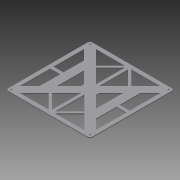
# Autodesk Inventor part: piastra_superiore_y
Saved by Autodesk Inventor 2014 SP1 (Build 180222100, 222)
## iProperties
Created: 2015-04-08
Part Number: piastra_superiore_y
Material: Generic
Document SubType Name: Modeling
Designer: Giorgio Nuzzo
Density: 1 g/cm^3
Appearance: Default
Author: Giorgio Nuzzo
Autodesk Inventor part; units mm, degrees
(part 1 of 3)
ref_plane "YZ Plane" through (0, 0, 0) normal (1, 0, 0) x (0, 1, 0)
ref_plane "XZ Plane" through (0, 0, 0) normal (0, 1, 0) x (-1, 0, 0)
ref_plane "XY Plane" through (0, 0, 0) normal (0, 0, 1) x (1, 0, 0)
sketch "Sketch1" plane through (0, 0, 0) normal (0, 0, 1) x (1, 0, 0)
  spline S0 degree 3 poles (-107.5002, -101.5001) (-107.5002, -104.8136) (-104.8138, -107.5001) (-101.5, -107.5001) knots 0 0 0 0 1 1 1 1
  line L0 (-107.5002, -101.5001) -> (-107.5002, -104.8136) construction
  line L1 (-107.5002, -104.8136) -> (-104.8138, -107.5001) construction
  line L2 (-104.8138, -107.5001) -> (-101.5, -107.5001) construction
  line L3 (-101.5, -107.5001) -> (101.5, -107.5001)
  spline S1 degree 3 poles (101.5, -107.5001) (104.8135, -107.5001) (107.5, -104.8136) (107.5, -101.5001) knots 2 2 2 2 3 3 3 3
  line L4 (101.5, -107.5001) -> (104.8135, -107.5001) construction
  line L5 (104.8135, -107.5001) -> (107.5, -104.8136) construction
  line L6 (107.5, -104.8136) -> (107.5, -101.5001) construction
  line L7 (107.5, -101.5001) -> (107.5, 101.5001)
  spline S2 degree 3 poles (107.5, 101.5001) (107.5, 104.8138) (104.8135, 107.5001) (101.5, 107.5001) (101.5, 107.5001) (-101.5, 107.5001) (-101.5, 107.5001) (-104.8138, 107.5001) (-107.5002, 104.8138) (-107.5002, 101.5001) (-107.5002, 101.5001) (-107.5002, -101.2971) (-107.5002, -101.5001) knots 4 4 4 4 5 5 5 6 6 6 7 7 7 8 8 8 8
  line L8 (107.5, 101.5001) -> (107.5, 104.8138) construction
  line L9 (107.5, 104.8138) -> (104.8135, 107.5001) construction
  line L10 (104.8135, 107.5001) -> (101.5, 107.5001) construction
  line L11 (101.5, 107.5001) -> (101.5, 107.5001) construction
  line L12 (101.5, 107.5001) -> (-101.5, 107.5001) construction
  line L13 (-101.5, 107.5001) -> (-101.5, 107.5001) construction
  line L14 (-101.5, 107.5001) -> (-104.8138, 107.5001) construction
  line L15 (-104.8138, 107.5001) -> (-107.5002, 104.8138) construction
  line L16 (-107.5002, 104.8138) -> (-107.5002, 101.5001) construction
  line L17 (-107.5002, 101.5001) -> (-107.5002, 101.5001) construction
  line L18 (-107.5002, 101.5001) -> (-107.5002, -101.5001) construction
  line L19 (-107.5002, -101.5001) -> (-107.5002, -101.5001) construction
  line L20 (4.9998, -107.5001) -> (84.925, -107.5001)
  line L21 (-97.4892, 82.4918) -> (-72.0064, 57.0089)
  line L22 (-72.0064, 57.0089) -> (-72.0064, 3.9999)
  line L23 (-72.0064, 3.9999) -> (-97.4892, 4.0106)
  line L24 (-97.4892, 4.0106) -> (-97.4892, 82.4918)
  line L25 (-97.4892, -82.4901) -> (-72.0064, -57.007)
  line L26 (-72.0064, -57.007) -> (-72.0064, -4.0001)
  line L27 (-72.0064, -4.0001) -> (-97.4892, -4.0001)
  line L28 (-97.4892, -4.0001) -> (-97.4892, -82.4901)
  line L29 (-19.4509, 4.4535) -> (-50.0063, 35.0089)
  line L30 (-50.0063, 35.0089) -> (-50.0063, -4.0001)
  line L31 (-50.0063, -4.0001) -> (-50.0063, -35.007)
  line L32 (-50.0063, -35.007) -> (-49.8928, -34.8936)
  line L33 (-49.8928, -34.8936) -> (-32.5743, -17.5752)
  line L34 (-32.5743, -17.5752) -> (-19.4509, -4.4518)
  line L35 (-19.4509, -4.4518) -> (-19.4509, -4.0001)
  line L36 (-19.4509, -4.0001) -> (-19.4509, 3.9999)
  line L37 (-19.4509, 3.9999) -> (-19.4509, 4.4535)
  line L38 (-3.9981, 93.318) -> (-3.9981, 18.9804)
  line L39 (-3.9981, 18.9804) -> (-32.5743, 47.5568)
  line L40 (-32.5743, 47.5568) -> (-41.1669, 56.1492)
  line L41 (-41.1669, 56.1492) -> (-3.9981, 93.318)
  line L42 (4.0017, 93.294) -> (41.1371, 56.1588)
  line L43 (41.1371, 56.1588) -> (4.0017, 19.0236)
  line L44 (4.0017, 19.0236) -> (4.0017, 93.294)
  line L45 (45.3797, 60.4015) -> (82.4876, 97.5093)
  line L46 (82.4876, 97.5093) -> (8.2719, 97.5093)
  line L47 (8.2719, 97.5093) -> (45.3797, 60.4015)
  line L48 (-8.2921, 97.5093) -> (-45.4095, 60.3918)
  line L49 (-45.4095, 60.3918) -> (-49.8928, 64.8751)
  line L50 (-49.8928, 64.8751) -> (-82.5268, 97.5093)
  line L51 (-82.5268, 97.5093) -> (-8.2921, 97.5093)
  line L52 (19.4003, -4.4028) -> (19.4003, -4.0001)
  line L53 (19.4003, -4.0001) -> (19.4003, 3.9999)
  line L54 (19.4003, 3.9999) -> (19.4003, 4.4423)
  line L55 (19.4003, 4.4423) -> (50.0062, 35.0482)
  line L56 (50.0062, 35.0482) -> (50.0062, 3.9999)
  line L57 (50.0062, 3.9999) -> (50.0062, -4.0001)
  line L58 (50.0062, -4.0001) -> (50.0062, -35.0087)
  line L59 (50.0062, -35.0087) -> (19.4003, -4.4028)
  line L60 (97.4996, 82.5416) -> (72.0062, 57.0482)
  line L61 (72.0062, 57.0482) -> (72.0062, 3.9999)
  line L62 (72.0062, 3.9999) -> (97.4996, 3.9999)
  line L63 (97.4996, 3.9999) -> (97.4996, 82.5416)
  line L64 (97.4996, -82.5021) -> (72.0062, -57.0088)
  line L65 (72.0062, -57.0088) -> (72.0062, -4.0001)
  line L66 (72.0062, -4.0001) -> (97.4996, -4.0001)
  line L67 (97.4996, -4.0001) -> (97.4996, -82.5021)
  line L68 (-8.2921, -97.3935) -> (-45.4095, -60.2761)
  line L69 (-45.4095, -60.2761) -> (-49.8928, -64.7595)
  line L70 (-49.8928, -64.7595) -> (-82.5268, -97.3935)
  line L71 (-82.5268, -97.3935) -> (-8.2921, -97.3935)
  line L72 (-3.9981, -93.2022) -> (-3.9981, -18.8647)
  line L73 (-3.9981, -18.8647) -> (-32.5743, -47.441)
  line L74 (-32.5743, -47.441) -> (-41.1669, -56.0334)
  line L75 (-41.1669, -56.0334) -> (-3.9981, -93.2022)
  line L76 (4.0017, -93.1785) -> (41.1371, -56.0431)
  line L77 (41.1371, -56.0431) -> (4.0017, -18.9081)
  line L78 (4.0017, -18.9081) -> (4.0017, -93.1785)
  line L79 (45.3797, -60.2857) -> (82.4876, -97.3935)
  line L80 (82.4876, -97.3935) -> (8.2719, -97.3935)
  line L81 (8.2719, -97.3935) -> (45.3797, -60.2857)
  line L82 (-102.0988, 0.0012) -> (-102.0907, 0.1648)
  line L83 (-102.0907, 0.1648) -> (-102.0664, 0.3237)
  line L84 (-102.0664, 0.3237) -> (-102.0269, 0.477)
  line L85 (-102.0269, 0.477) -> (-101.9732, 0.6241)
  line L86 (-101.9732, 0.6241) -> (-101.9057, 0.7639)
  line L87 (-101.9057, 0.7639) -> (-101.8256, 0.8957)
  line L88 (-101.8256, 0.8957) -> (-101.6302, 1.1326)
  line L89 (-101.6302, 1.1326) -> (-101.3934, 1.3279)
  line L90 (-101.3934, 1.3279) -> (-101.2614, 1.4082)
  line L91 (-101.2614, 1.4082) -> (-101.1216, 1.4755)
  line L92 (-101.1216, 1.4755) -> (-100.9746, 1.5293)
  line L93 (-100.9746, 1.5293) -> (-100.8213, 1.5687)
  line L94 (-100.8213, 1.5687) -> (-100.6625, 1.593)
  line L95 (-100.6625, 1.593) -> (-100.4989, 1.6013)
  line L96 (-100.4989, 1.6013) -> (-100.3352, 1.593)
  line L97 (-100.3352, 1.593) -> (-100.1764, 1.5687)
  line L98 (-100.1764, 1.5687) -> (-100.0231, 1.5293)
  line L99 (-100.0231, 1.5293) -> (-99.876, 1.4755)
  line L100 (-99.876, 1.4755) -> (-99.7361, 1.4082)
  line L101 (-99.7361, 1.4082) -> (-99.6043, 1.3279)
  line L102 (-99.6043, 1.3279) -> (-99.3675, 1.1326)
  line L103 (-99.3675, 1.1326) -> (-99.1722, 0.8957)
  line L104 (-99.1722, 0.8957) -> (-99.0919, 0.7639)
  line L105 (-99.0919, 0.7639) -> (-99.0245, 0.6241)
  line L106 (-99.0245, 0.6241) -> (-98.9708, 0.477)
  line L107 (-98.9708, 0.477) -> (-98.9313, 0.3237)
  line L108 (-98.9313, 0.3237) -> (-98.9071, 0.1648)
  line L109 (-98.9071, 0.1648) -> (-98.8988, 0.0012)
  line L110 (-98.8988, 0.0012) -> (-98.9071, -0.1624)
  line L111 (-98.9071, -0.1624) -> (-98.9313, -0.3213)
  line L112 (-98.9313, -0.3213) -> (-98.9708, -0.4747)
  line L113 (-98.9708, -0.4747) -> (-99.0245, -0.6215)
  line L114 (-99.0245, -0.6215) -> (-99.0919, -0.7614)
  line L115 (-99.0919, -0.7614) -> (-99.1722, -0.8933)
  line L116 (-99.1722, -0.8933) -> (-99.3675, -1.13)
  line L117 (-99.3675, -1.13) -> (-99.6043, -1.3257)
  line L118 (-99.6043, -1.3257) -> (-99.7361, -1.4056)
  line L119 (-99.7361, -1.4056) -> (-99.876, -1.4731)
  line L120 (-99.876, -1.4731) -> (-100.0231, -1.5269)
  line L121 (-100.0231, -1.5269) -> (-100.1764, -1.5661)
  line L122 (-100.1764, -1.5661) -> (-100.3352, -1.5906)
  line L123 (-100.3352, -1.5906) -> (-100.4989, -1.5989)
  line L124 (-100.4989, -1.5989) -> (-100.6625, -1.5906)
  line L125 (-100.6625, -1.5906) -> (-100.8213, -1.5661)
  line L126 (-100.8213, -1.5661) -> (-100.9746, -1.5269)
  line L127 (-100.9746, -1.5269) -> (-101.1216, -1.4731)
  line L128 (-101.1216, -1.4731) -> (-101.2614, -1.4056)
  line L129 (-101.2614, -1.4056) -> (-101.3934, -1.3257)
  line L130 (-101.3934, -1.3257) -> (-101.6302, -1.13)
  line L131 (-101.6302, -1.13) -> (-101.8256, -0.8933)
  line L132 (-101.8256, -0.8933) -> (-101.9057, -0.7614)
  line L133 (-101.9057, -0.7614) -> (-101.9732, -0.6215)
  line L134 (-101.9732, -0.6215) -> (-102.0269, -0.4747)
  line L135 (-102.0269, -0.4747) -> (-102.0664, -0.3213)
  line L136 (-102.0664, -0.3213) -> (-102.0907, -0.1624)
  line L137 (-102.0907, -0.1624) -> (-102.0988, 0.0012)
  line L138 (98.899, 0.0012) -> (98.9072, 0.1648)
  line L139 (98.9072, 0.1648) -> (98.9317, 0.3237)
  line L140 (98.9317, 0.3237) -> (98.971, 0.477)
  line L141 (98.971, 0.477) -> (99.0247, 0.6241)
  line L142 (99.0247, 0.6241) -> (99.0922, 0.7639)
  line L143 (99.0922, 0.7639) -> (99.1725, 0.8957)
  line L144 (99.1725, 0.8957) -> (99.3678, 1.1326)
  line L145 (99.3678, 1.1326) -> (99.6045, 1.3279)
  line L146 (99.6045, 1.3279) -> (99.7365, 1.4082)
  line L147 (99.7365, 1.4082) -> (99.8763, 1.4755)
  line L148 (99.8763, 1.4755) -> (100.0234, 1.5293)
  line L149 (100.0234, 1.5293) -> (100.1767, 1.5687)
  line L150 (100.1767, 1.5687) -> (100.3356, 1.593)
  line L151 (100.3356, 1.593) -> (100.4992, 1.6013)
  line L152 (100.4992, 1.6013) -> (100.6628, 1.593)
  line L153 (100.6628, 1.593) -> (100.8217, 1.5687)
  line L154 (100.8217, 1.5687) -> (100.975, 1.5293)
  line L155 (100.975, 1.5293) -> (101.1217, 1.4755)
  line L156 (101.1217, 1.4755) -> (101.2616, 1.4082)
  line L157 (101.2616, 1.4082) -> (101.3936, 1.3279)
  line L158 (101.3936, 1.3279) -> (101.6306, 1.1326)
  line L159 (101.6306, 1.1326) -> (101.8259, 0.8957)
  line L160 (101.8259, 0.8957) -> (101.9058, 0.7639)
  line L161 (101.9058, 0.7639) -> (101.9734, 0.6241)
  line L162 (101.9734, 0.6241) -> (102.0271, 0.477)
  line L163 (102.0271, 0.477) -> (102.0667, 0.3237)
  line L164 (102.0667, 0.3237) -> (102.0908, 0.1648)
  line L165 (102.0908, 0.1648) -> (102.0991, 0.0012)
  line L166 (102.0991, 0.0012) -> (102.0908, -0.1624)
  line L167 (102.0908, -0.1624) -> (102.0667, -0.3213)
  line L168 (102.0667, -0.3213) -> (102.0271, -0.4747)
  line L169 (102.0271, -0.4747) -> (101.9734, -0.6215)
  line L170 (101.9734, -0.6215) -> (101.9058, -0.7614)
  line L171 (101.9058, -0.7614) -> (101.8259, -0.8933)
  line L172 (101.8259, -0.8933) -> (101.6306, -1.13)
  line L173 (101.6306, -1.13) -> (101.3936, -1.3257)
  line L174 (101.3936, -1.3257) -> (101.2616, -1.4056)
  line L175 (101.2616, -1.4056) -> (101.1217, -1.4731)
  line L176 (101.1217, -1.4731) -> (100.975, -1.5269)
  line L177 (100.975, -1.5269) -> (100.8217, -1.5661)
  line L178 (100.8217, -1.5661) -> (100.6628, -1.5906)
  line L179 (100.6628, -1.5906) -> (100.4992, -1.5989)
  line L180 (100.4992, -1.5989) -> (100.3356, -1.5906)
  line L181 (100.3356, -1.5906) -> (100.1767, -1.5661)
  line L182 (100.1767, -1.5661) -> (100.0234, -1.5269)
  line L183 (100.0234, -1.5269) -> (99.8763, -1.4731)
  line L184 (99.8763, -1.4731) -> (99.7365, -1.4056)
  line L185 (99.7365, -1.4056) -> (99.6045, -1.3257)
  line L186 (99.6045, -1.3257) -> (99.3678, -1.13)
  line L187 (99.3678, -1.13) -> (99.1725, -0.8933)
  line L188 (99.1725, -0.8933) -> (99.0922, -0.7614)
  line L189 (99.0922, -0.7614) -> (99.0247, -0.6215)
  line L190 (99.0247, -0.6215) -> (98.971, -0.4747)
  line L191 (98.971, -0.4747) -> (98.9317, -0.3213)
  line L192 (98.9317, -0.3213) -> (98.9072, -0.1624)
  line L193 (98.9072, -0.1624) -> (98.899, 0.0012)
  line L194 (-1.6014, 100.496) -> (-1.5931, 100.6595)
  line L195 (-1.5931, 100.6595) -> (-1.5688, 100.8185)
  line L196 (-1.5688, 100.8185) -> (-1.5294, 100.9718)
  line L197 (-1.5294, 100.9718) -> (-1.4756, 101.1187)
  line L198 (-1.4756, 101.1187) -> (-1.4083, 101.2586)
  line L199 (-1.4083, 101.2586) -> (-1.328, 101.3905)
  line L200 (-1.328, 101.3905) -> (-1.1327, 101.6274)
  line L201 (-1.1327, 101.6274) -> (-0.8958, 101.8227)
  line L202 (-0.8958, 101.8227) -> (-0.764, 101.9028)
  line L203 (-0.764, 101.9028) -> (-0.6242, 101.9702)
  line L204 (-0.6242, 101.9702) -> (-0.4771, 102.0241)
  line L205 (-0.4771, 102.0241) -> (-0.3238, 102.0634)
  line L206 (-0.3238, 102.0634) -> (-0.1649, 102.0877)
  line L207 (-0.1649, 102.0877) -> (-0.0013, 102.0959)
  line L208 (-0.0013, 102.0959) -> (0.1622, 102.0877)
  line L209 (0.1622, 102.0877) -> (0.321, 102.0634)
  line L210 (0.321, 102.0634) -> (0.4746, 102.0241)
  line L211 (0.4746, 102.0241) -> (0.6214, 101.9702)
  line L212 (0.6214, 101.9702) -> (0.7613, 101.9028)
  line L213 (0.7613, 101.9028) -> (0.8932, 101.8227)
  line L214 (0.8932, 101.8227) -> (1.1299, 101.6274)
  line L215 (1.1299, 101.6274) -> (1.3256, 101.3905)
  line L216 (1.3256, 101.3905) -> (1.4055, 101.2586)
  line L217 (1.4055, 101.2586) -> (1.473, 101.1187)
  line L218 (1.473, 101.1187) -> (1.5268, 100.9718)
  line L219 (1.5268, 100.9718) -> (1.5661, 100.8185)
  line L220 (1.5661, 100.8185) -> (1.5905, 100.6595)
  line L221 (1.5905, 100.6595) -> (1.5988, 100.496)
  line L222 (1.5988, 100.496) -> (1.5905, 100.3324)
  line L223 (1.5905, 100.3324) -> (1.5661, 100.1736)
  line L224 (1.5661, 100.1736) -> (1.5268, 100.0201)
  line L225 (1.5268, 100.0201) -> (1.473, 99.8731)
  line L226 (1.473, 99.8731) -> (1.4055, 99.7333)
  line L227 (1.4055, 99.7333) -> (1.3256, 99.6013)
  line L228 (1.3256, 99.6013) -> (1.1299, 99.3646)
  line L229 (1.1299, 99.3646) -> (0.8932, 99.1691)
  line L230 (0.8932, 99.1691) -> (0.7613, 99.089)
  line L231 (0.7613, 99.089) -> (0.6214, 99.0217)
  line L232 (0.6214, 99.0217) -> (0.4746, 98.9679)
  line L233 (0.4746, 98.9679) -> (0.321, 98.9285)
  line L234 (0.321, 98.9285) -> (0.1622, 98.9042)
  line L235 (0.1622, 98.9042) -> (-0.0013, 98.8959)
  line L236 (-0.0013, 98.8959) -> (-0.1649, 98.9042)
  line L237 (-0.1649, 98.9042) -> (-0.3238, 98.9285)
  line L238 (-0.3238, 98.9285) -> (-0.4771, 98.9679)
  line L239 (-0.4771, 98.9679) -> (-0.6242, 99.0217)
  line L240 (-0.6242, 99.0217) -> (-0.764, 99.089)
  line L241 (-0.764, 99.089) -> (-0.8958, 99.1691)
  line L242 (-0.8958, 99.1691) -> (-1.1327, 99.3646)
  line L243 (-1.1327, 99.3646) -> (-1.328, 99.6013)
  line L244 (-1.328, 99.6013) -> (-1.4083, 99.7333)
  line L245 (-1.4083, 99.7333) -> (-1.4756, 99.8731)
  line L246 (-1.4756, 99.8731) -> (-1.5294, 100.0201)
  line L247 (-1.5294, 100.0201) -> (-1.5688, 100.1736)
  line L248 (-1.5688, 100.1736) -> (-1.5931, 100.3324)
  line L249 (-1.5931, 100.3324) -> (-1.6014, 100.496)
  line L250 (-1.6014, -100.4996) -> (-1.5931, -100.336)
  line L251 (-1.5931, -100.336) -> (-1.5688, -100.1772)
  line L252 (-1.5688, -100.1772) -> (-1.5294, -100.0239)
  line L253 (-1.5294, -100.0239) -> (-1.4756, -99.8768)
  line L254 (-1.4756, -99.8768) -> (-1.4083, -99.7369)
  line L255 (-1.4083, -99.7369) -> (-1.328, -99.6049)
  line L256 (-1.328, -99.6049) -> (-1.1327, -99.3683)
  line L257 (-1.1327, -99.3683) -> (-0.8958, -99.1729)
  line L258 (-0.8958, -99.1729) -> (-0.764, -99.0927)
  line L259 (-0.764, -99.0927) -> (-0.6242, -99.0255)
  line L260 (-0.6242, -99.0255) -> (-0.4771, -98.9717)
  line L261 (-0.4771, -98.9717) -> (-0.3238, -98.9321)
  line L262 (-0.3238, -98.9321) -> (-0.1649, -98.908)
  line L263 (-0.1649, -98.908) -> (-0.0013, -98.8997)
  line L264 (-0.0013, -98.8997) -> (0.1622, -98.908)
  line L265 (0.1622, -98.908) -> (0.321, -98.9321)
  line L266 (0.321, -98.9321) -> (0.4746, -98.9717)
  line L267 (0.4746, -98.9717) -> (0.6214, -99.0255)
  line L268 (0.6214, -99.0255) -> (0.7613, -99.0927)
  line L269 (0.7613, -99.0927) -> (0.8932, -99.1729)
  line L270 (0.8932, -99.1729) -> (1.1299, -99.3683)
  line L271 (1.1299, -99.3683) -> (1.3256, -99.6049)
  line L272 (1.3256, -99.6049) -> (1.4055, -99.7369)
  line L273 (1.4055, -99.7369) -> (1.473, -99.8768)
  line L274 (1.473, -99.8768) -> (1.5268, -100.0239)
  line L275 (1.5268, -100.0239) -> (1.5661, -100.1772)
  line L276 (1.5661, -100.1772) -> (1.5905, -100.336)
  line L277 (1.5905, -100.336) -> (1.5988, -100.4996)
  line L278 (1.5988, -100.4996) -> (1.5905, -100.6633)
  line L279 (1.5905, -100.6633) -> (1.5661, -100.8221)
  line L280 (1.5661, -100.8221) -> (1.5268, -100.9754)
  line L281 (1.5268, -100.9754) -> (1.473, -101.1225)
  line L282 (1.473, -101.1225) -> (1.4055, -101.2624)
  line L283 (1.4055, -101.2624) -> (1.3256, -101.3943)
  line L284 (1.3256, -101.3943) -> (1.1299, -101.631)
  line L285 (1.1299, -101.631) -> (0.8932, -101.8263)
  line L286 (0.8932, -101.8263) -> (0.7613, -101.9066)
  line L287 (0.7613, -101.9066) -> (0.6214, -101.9738)
  line L288 (0.6214, -101.9738) -> (0.4746, -102.0279)
  line L289 (0.4746, -102.0279) -> (0.321, -102.0672)
  line L290 (0.321, -102.0672) -> (0.1622, -102.0913)
  line L291 (0.1622, -102.0913) -> (-0.0013, -102.0995)
  line L292 (-0.0013, -102.0995) -> (-0.1649, -102.0913)
  line L293 (-0.1649, -102.0913) -> (-0.3238, -102.0672)
  line L294 (-0.3238, -102.0672) -> (-0.4771, -102.0279)
  line L295 (-0.4771, -102.0279) -> (-0.6242, -101.9738)
  line L296 (-0.6242, -101.9738) -> (-0.764, -101.9066)
  line L297 (-0.764, -101.9066) -> (-0.8958, -101.8263)
  line L298 (-0.8958, -101.8263) -> (-1.1327, -101.631)
  line L299 (-1.1327, -101.631) -> (-1.328, -101.3943)
  line L300 (-1.328, -101.3943) -> (-1.4083, -101.2624)
  line L301 (-1.4083, -101.2624) -> (-1.4756, -101.1225)
  line L302 (-1.4756, -101.1225) -> (-1.5294, -100.9754)
  line L303 (-1.5294, -100.9754) -> (-1.5688, -100.8221)
  line L304 (-1.5688, -100.8221) -> (-1.5931, -100.6633)
  line L305 (-1.5931, -100.6633) -> (-1.6014, -100.4996)
  line L306 (98.899, -100.5) -> (98.9072, -100.3363)
  line L307 (98.9072, -100.3363) -> (98.9313, -100.1775)
  line L308 (98.9313, -100.1775) -> (98.971, -100.0242)
  line L309 (98.971, -100.0242) -> (99.0247, -99.8771)
  line L310 (99.0247, -99.8771) -> (99.0919, -99.7372)
  line L311 (99.0919, -99.7372) -> (99.1722, -99.6053)
  line L312 (99.1722, -99.6053) -> (99.3675, -99.3686)
  line L313 (99.3675, -99.3686) -> (99.6045, -99.1733)
  line L314 (99.6045, -99.1733) -> (99.7361, -99.093)
  line L315 (99.7361, -99.093) -> (99.876, -99.0258)
  line L316 (99.876, -99.0258) -> (100.0231, -98.9721)
  line L317 (100.0231, -98.9721) -> (100.1764, -98.9325)
  line L318 (100.1764, -98.9325) -> (100.3352, -98.9083)
  line L319 (100.3352, -98.9083) -> (100.4989, -98.9001)
  line L320 (100.4989, -98.9001) -> (100.6625, -98.9083)
  line L321 (100.6625, -98.9083) -> (100.8213, -98.9325)
  line L322 (100.8213, -98.9325) -> (100.9746, -98.9721)
  line L323 (100.9746, -98.9721) -> (101.1217, -99.0258)
  line L324 (101.1217, -99.0258) -> (101.2616, -99.093)
  line L325 (101.2616, -99.093) -> (101.3936, -99.1733)
  line L326 (101.3936, -99.1733) -> (101.6302, -99.3686)
  line L327 (101.6302, -99.3686) -> (101.8256, -99.6053)
  line L328 (101.8256, -99.6053) -> (101.9058, -99.7372)
  line L329 (101.9058, -99.7372) -> (101.973, -99.8771)
  line L330 (101.973, -99.8771) -> (102.0271, -100.0242)
  line L331 (102.0271, -100.0242) -> (102.0664, -100.1775)
  line L332 (102.0664, -100.1775) -> (102.0905, -100.3363)
  line L333 (102.0905, -100.3363) -> (102.0988, -100.5)
  line L334 (102.0988, -100.5) -> (102.0905, -100.6636)
  line L335 (102.0905, -100.6636) -> (102.0664, -100.8224)
  line L336 (102.0664, -100.8224) -> (102.0271, -100.9757)
  line L337 (102.0271, -100.9757) -> (101.973, -101.1229)
  line L338 (101.973, -101.1229) -> (101.9058, -101.2627)
  line L339 (101.9058, -101.2627) -> (101.8256, -101.3947)
  line L340 (101.8256, -101.3947) -> (101.6302, -101.6314)
  line L341 (101.6302, -101.6314) -> (101.3936, -101.8267)
  line L342 (101.3936, -101.8267) -> (101.2616, -101.907)
  line L343 (101.2616, -101.907) -> (101.1217, -101.9741)
  line L344 (101.1217, -101.9741) -> (100.9746, -102.0282)
  line L345 (100.9746, -102.0282) -> (100.8213, -102.0675)
  line L346 (100.8213, -102.0675) -> (100.6625, -102.0916)
  line L347 (100.6625, -102.0916) -> (100.4989, -102.0999)
  line L348 (100.4989, -102.0999) -> (100.3352, -102.0916)
  line L349 (100.3352, -102.0916) -> (100.1764, -102.0675)
  line L350 (100.1764, -102.0675) -> (100.0231, -102.0282)
  line L351 (100.0231, -102.0282) -> (99.876, -101.9741)
  line L352 (99.876, -101.9741) -> (99.7361, -101.907)
  line L353 (99.7361, -101.907) -> (99.6045, -101.8267)
  line L354 (99.6045, -101.8267) -> (99.3675, -101.6314)
  line L355 (99.3675, -101.6314) -> (99.1722, -101.3947)
  line L356 (99.1722, -101.3947) -> (99.0919, -101.2627)
  line L357 (99.0919, -101.2627) -> (99.0247, -101.1229)
  line L358 (99.0247, -101.1229) -> (98.971, -100.9757)
  line L359 (98.971, -100.9757) -> (98.9313, -100.8224)
  line L360 (98.9313, -100.8224) -> (98.9072, -100.6636)
  line L361 (98.9072, -100.6636) -> (98.899, -100.5)
  line L362 (-102.1177, -100.4983) -> (-102.1094, -100.3346)
  line L363 (-102.1094, -100.3346) -> (-102.0852, -100.1758)
  line L364 (-102.0852, -100.1758) -> (-102.0457, -100.0225)
  line L365 (-102.0457, -100.0225) -> (-101.992, -99.8754)
  line L366 (-101.992, -99.8754) -> (-101.9246, -99.7355)
  line L367 (-101.9246, -99.7355) -> (-101.8443, -99.6036)
  line L368 (-101.8443, -99.6036) -> (-101.649, -99.3669)
  line L369 (-101.649, -99.3669) -> (-101.4122, -99.1716)
  line L370 (-101.4122, -99.1716) -> (-101.2804, -99.0913)
  line L371 (-101.2804, -99.0913) -> (-101.1405, -99.0241)
  line L372 (-101.1405, -99.0241) -> (-100.9934, -98.97)
  line L373 (-100.9934, -98.97) -> (-100.8401, -98.9307)
  line L374 (-100.8401, -98.9307) -> (-100.6813, -98.9066)
  line L375 (-100.6813, -98.9066) -> (-100.5176, -98.8984)
  line L376 (-100.5176, -98.8984) -> (-100.354, -98.9066)
  line L377 (-100.354, -98.9066) -> (-100.1952, -98.9307)
  line L378 (-100.1952, -98.9307) -> (-100.0419, -98.97)
  line L379 (-100.0419, -98.97) -> (-99.8949, -99.0241)
  line L380 (-99.8949, -99.0241) -> (-99.7551, -99.0913)
  line L381 (-99.7551, -99.0913) -> (-99.6231, -99.1716)
  line L382 (-99.6231, -99.1716) -> (-99.3863, -99.3669)
  line L383 (-99.3863, -99.3669) -> (-99.1909, -99.6036)
  line L384 (-99.1909, -99.6036) -> (-99.1108, -99.7355)
  line L385 (-99.1108, -99.7355) -> (-99.0433, -99.8754)
  line L386 (-99.0433, -99.8754) -> (-98.9896, -100.0225)
  line L387 (-98.9896, -100.0225) -> (-98.9501, -100.1758)
  line L388 (-98.9501, -100.1758) -> (-98.9258, -100.3346)
  line L389 (-98.9258, -100.3346) -> (-98.9176, -100.4983)
  line L390 (-98.9176, -100.4983) -> (-98.9258, -100.6619)
  line L391 (-98.9258, -100.6619) -> (-98.9501, -100.8207)
  line L392 (-98.9501, -100.8207) -> (-98.9896, -100.974)
  line L393 (-98.9896, -100.974) -> (-99.0433, -101.1211)
  line L394 (-99.0433, -101.1211) -> (-99.1108, -101.261)
  line L395 (-99.1108, -101.261) -> (-99.1909, -101.3929)
  line L396 (-99.1909, -101.3929) -> (-99.3863, -101.6296)
  line L397 (-99.3863, -101.6296) -> (-99.6231, -101.825)
  line L398 (-99.6231, -101.825) -> (-99.7551, -101.9052)
  line L399 (-99.7551, -101.9052) -> (-99.8949, -101.9724)
  line L400 (-99.8949, -101.9724) -> (-100.0419, -102.0262)
  line L401 (-100.0419, -102.0262) -> (-100.1952, -102.0658)
  line L402 (-100.1952, -102.0658) -> (-100.354, -102.0899)
  line L403 (-100.354, -102.0899) -> (-100.5176, -102.0982)
  line L404 (-100.5176, -102.0982) -> (-100.6813, -102.0899)
  line L405 (-100.6813, -102.0899) -> (-100.8401, -102.0658)
  line L406 (-100.8401, -102.0658) -> (-100.9934, -102.0262)
  line L407 (-100.9934, -102.0262) -> (-101.1405, -101.9724)
  line L408 (-101.1405, -101.9724) -> (-101.2804, -101.9052)
  line L409 (-101.2804, -101.9052) -> (-101.4122, -101.825)
  line L410 (-101.4122, -101.825) -> (-101.649, -101.6296)
  line L411 (-101.649, -101.6296) -> (-101.8443, -101.3929)
  line L412 (-101.8443, -101.3929) -> (-101.9246, -101.261)
  line L413 (-101.9246, -101.261) -> (-101.992, -101.1211)
  line L414 (-101.992, -101.1211) -> (-102.0457, -100.974)
  line L415 (-102.0457, -100.974) -> (-102.0852, -100.8207)
  line L416 (-102.0852, -100.8207) -> (-102.1094, -100.6619)
  line L417 (-102.1094, -100.6619) -> (-102.1177, -100.4983)
  line L418 (-102.1001, 100.5) -> (-102.0919, 100.6636)
  line L419 (-102.0919, 100.6636) -> (-102.0676, 100.8224)
  line L420 (-102.0676, 100.8224) -> (-102.0281, 100.9757)
  line L421 (-102.0281, 100.9757) -> (-101.9744, 101.1229)
  line L422 (-101.9744, 101.1229) -> (-101.907, 101.2627)
  line L423 (-101.907, 101.2627) -> (-101.8268, 101.3945)
  line L424 (-101.8268, 101.3945) -> (-101.6314, 101.6314)
  line L425 (-101.6314, 101.6314) -> (-101.3946, 101.8267)
  line L426 (-101.3946, 101.8267) -> (-101.2628, 101.907)
  line L427 (-101.2628, 101.907) -> (-101.1229, 101.9743)
  line L428 (-101.1229, 101.9743) -> (-100.9758, 102.0281)
  line L429 (-100.9758, 102.0281) -> (-100.8225, 102.0675)
  line L430 (-100.8225, 102.0675) -> (-100.6637, 102.0918)
  line L431 (-100.6637, 102.0918) -> (-100.5001, 102.1001)
  line L432 (-100.5001, 102.1001) -> (-100.3364, 102.0918)
  line L433 (-100.3364, 102.0918) -> (-100.1776, 102.0675)
  line L434 (-100.1776, 102.0675) -> (-100.0243, 102.0281)
  line L435 (-100.0243, 102.0281) -> (-99.8774, 101.9743)
  line L436 (-99.8774, 101.9743) -> (-99.7375, 101.907)
  line L437 (-99.7375, 101.907) -> (-99.6055, 101.8267)
  line L438 (-99.6055, 101.8267) -> (-99.3687, 101.6314)
  line L439 (-99.3687, 101.6314) -> (-99.1734, 101.3945)
  line L440 (-99.1734, 101.3945) -> (-99.0933, 101.2627)
  line L441 (-99.0933, 101.2627) -> (-99.0257, 101.1229)
  line L442 (-99.0257, 101.1229) -> (-98.972, 100.9757)
  line L443 (-98.972, 100.9757) -> (-98.9325, 100.8224)
  line L444 (-98.9325, 100.8224) -> (-98.9084, 100.6636)
  line L445 (-98.9084, 100.6636) -> (-98.9002, 100.5)
  line L446 (-98.9002, 100.5) -> (-98.9084, 100.3363)
  line L447 (-98.9084, 100.3363) -> (-98.9325, 100.1775)
  line L448 (-98.9325, 100.1775) -> (-98.972, 100.0242)
  line L449 (-98.972, 100.0242) -> (-99.0257, 99.8773)
  line L450 (-99.0257, 99.8773) -> (-99.0933, 99.7374)
  line L451 (-99.0933, 99.7374) -> (-99.1734, 99.6055)
  line L452 (-99.1734, 99.6055) -> (-99.3687, 99.3686)
  line L453 (-99.3687, 99.3686) -> (-99.6055, 99.1733)
  line L454 (-99.6055, 99.1733) -> (-99.7375, 99.0932)
  line L455 (-99.7375, 99.0932) -> (-99.8774, 99.0258)
  line L456 (-99.8774, 99.0258) -> (-100.0243, 98.9719)
  line L457 (-100.0243, 98.9719) -> (-100.1776, 98.9325)
  line L458 (-100.1776, 98.9325) -> (-100.3364, 98.9083)
  line L459 (-100.3364, 98.9083) -> (-100.5001, 98.9001)
  line L460 (-100.5001, 98.9001) -> (-100.6637, 98.9083)
  line L461 (-100.6637, 98.9083) -> (-100.8225, 98.9325)
  line L462 (-100.8225, 98.9325) -> (-100.9758, 98.9719)
  line L463 (-100.9758, 98.9719) -> (-101.1229, 99.0258)
  line L464 (-101.1229, 99.0258) -> (-101.2628, 99.0932)
  line L465 (-101.2628, 99.0932) -> (-101.3946, 99.1733)
  line L466 (-101.3946, 99.1733) -> (-101.6314, 99.3686)
  line L467 (-101.6314, 99.3686) -> (-101.8268, 99.6055)
  line L468 (-101.8268, 99.6055) -> (-101.907, 99.7374)
  line L469 (-101.907, 99.7374) -> (-101.9744, 99.8773)
  line L470 (-101.9744, 99.8773) -> (-102.0281, 100.0242)
  line L471 (-102.0281, 100.0242) -> (-102.0676, 100.1775)
  line L472 (-102.0676, 100.1775) -> (-102.0919, 100.3363)
  line L473 (-102.0919, 100.3363) -> (-102.1001, 100.5)
  line L474 (98.9003, 100.5) -> (98.9086, 100.6636)
  line L475 (98.9086, 100.6636) -> (98.9327, 100.8224)
  line L476 (98.9327, 100.8224) -> (98.972, 100.9757)
  line L477 (98.972, 100.9757) -> (99.0261, 101.1229)
  line L478 (99.0261, 101.1229) -> (99.0933, 101.2627)
  line L479 (99.0933, 101.2627) -> (99.1735, 101.3945)
  line L480 (99.1735, 101.3945) -> (99.3689, 101.6314)
  line L481 (99.3689, 101.6314) -> (99.6055, 101.8267)
  line L482 (99.6055, 101.8267) -> (99.7375, 101.907)
  line L483 (99.7375, 101.907) -> (99.8774, 101.9743)
  line L484 (99.8774, 101.9743) -> (100.0245, 102.0281)
  line L485 (100.0245, 102.0281) -> (100.1778, 102.0675)
  line L486 (100.1778, 102.0675) -> (100.3366, 102.0918)
  line L487 (100.3366, 102.0918) -> (100.5002, 102.1001)
  line L488 (100.5002, 102.1001) -> (100.6639, 102.0918)
  line L489 (100.6639, 102.0918) -> (100.8227, 102.0675)
  line L490 (100.8227, 102.0675) -> (100.976, 102.0281)
  line L491 (100.976, 102.0281) -> (101.1231, 101.9743)
  line L492 (101.1231, 101.9743) -> (101.263, 101.907)
  line L493 (101.263, 101.907) -> (101.3949, 101.8267)
  line L494 (101.3949, 101.8267) -> (101.6316, 101.6314)
  line L495 (101.6316, 101.6314) -> (101.8269, 101.3945)
  line L496 (101.8269, 101.3945) -> (101.9072, 101.2627)
  line L497 (101.9072, 101.2627) -> (101.9744, 101.1229)
  line L498 (101.9744, 101.1229) -> (102.0281, 100.9757)
  line L499 (102.0281, 100.9757) -> (102.0678, 100.8224)
  line L500 (102.0678, 100.8224) -> (102.0919, 100.6636)
  line L501 (102.0919, 100.6636) -> (102.1001, 100.5)
  line L502 (102.1001, 100.5) -> (102.0919, 100.3363)
  line L503 (102.0919, 100.3363) -> (102.0678, 100.1775)
  line L504 (102.0678, 100.1775) -> (102.0281, 100.0242)
  line L505 (102.0281, 100.0242) -> (101.9744, 99.8773)
  line L506 (101.9744, 99.8773) -> (101.9072, 99.7374)
  line L507 (101.9072, 99.7374) -> (101.8269, 99.6055)
  line L508 (101.8269, 99.6055) -> (101.6316, 99.3686)
  line L509 (101.6316, 99.3686) -> (101.3949, 99.1733)
  line L510 (101.3949, 99.1733) -> (101.263, 99.0932)
  line L511 (101.263, 99.0932) -> (101.1231, 99.0258)
  line L512 (101.1231, 99.0258) -> (100.976, 98.9719)
  line L513 (100.976, 98.9719) -> (100.8227, 98.9325)
  line L514 (100.8227, 98.9325) -> (100.6639, 98.9083)
  line L515 (100.6639, 98.9083) -> (100.5002, 98.9001)
  line L516 (100.5002, 98.9001) -> (100.3366, 98.9083)
  line L517 (100.3366, 98.9083) -> (100.1778, 98.9325)
  line L518 (100.1778, 98.9325) -> (100.0245, 98.9719)
  line L519 (100.0245, 98.9719) -> (99.8774, 99.0258)
  line L520 (99.8774, 99.0258) -> (99.7375, 99.0932)
  line L521 (99.7375, 99.0932) -> (99.6055, 99.1733)
  line L522 (99.6055, 99.1733) -> (99.3689, 99.3686)
  line L523 (99.3689, 99.3686) -> (99.1735, 99.6055)
  line L524 (99.1735, 99.6055) -> (99.0933, 99.7374)
  line L525 (99.0933, 99.7374) -> (99.0261, 99.8773)
  line L526 (99.0261, 99.8773) -> (98.972, 100.0242)
  line L527 (98.972, 100.0242) -> (98.9327, 100.1775)
  line L528 (98.9327, 100.1775) -> (98.9086, 100.3363)
  line L529 (98.9086, 100.3363) -> (98.9003, 100.5)
  line L530 (76.8948, 78.513) -> (76.9031, 78.6767)
  line L531 (76.9031, 78.6767) -> (76.9272, 78.8355)
  line L532 (76.9272, 78.8355) -> (76.9668, 78.9888)
  line L533 (76.9668, 78.9888) -> (77.0205, 79.1359)
  line L534 (77.0205, 79.1359) -> (77.0877, 79.2758)
  line L535 (77.0877, 79.2758) -> (77.168, 79.4076)
  line L536 (77.168, 79.4076) -> (77.3633, 79.6444)
  line L537 (77.3633, 79.6444) -> (77.6, 79.8397)
  line L538 (77.6, 79.8397) -> (77.7319, 79.92)
  line L539 (77.7319, 79.92) -> (77.8718, 79.9874)
  line L540 (77.8718, 79.9874) -> (78.0189, 80.0411)
  line L541 (78.0189, 80.0411) -> (78.1722, 80.0806)
  line L542 (78.1722, 80.0806) -> (78.331, 80.1048)
  line L543 (78.331, 80.1048) -> (78.4947, 80.1131)
  line L544 (78.4947, 80.1131) -> (78.6583, 80.1048)
  line L545 (78.6583, 80.1048) -> (78.8172, 80.0806)
  line L546 (78.8172, 80.0806) -> (78.9705, 80.0411)
  line L547 (78.9705, 80.0411) -> (79.1176, 79.9874)
  line L548 (79.1176, 79.9874) -> (79.2574, 79.92)
  line L549 (79.2574, 79.92) -> (79.3894, 79.8397)
  line L550 (79.3894, 79.8397) -> (79.6261, 79.6444)
  line L551 (79.6261, 79.6444) -> (79.8214, 79.4076)
  line L552 (79.8214, 79.4076) -> (79.9017, 79.2758)
  line L553 (79.9017, 79.2758) -> (79.9688, 79.1359)
  line L554 (79.9688, 79.1359) -> (80.0226, 78.9888)
  line L555 (80.0226, 78.9888) -> (80.0622, 78.8355)
  line L556 (80.0622, 78.8355) -> (80.0863, 78.6767)
  line L557 (80.0863, 78.6767) -> (80.0946, 78.513)
  line L558 (80.0946, 78.513) -> (80.0863, 78.3494)
  line L559 (80.0863, 78.3494) -> (80.0622, 78.1906)
  line L560 (80.0622, 78.1906) -> (80.0226, 78.0373)
  line L561 (80.0226, 78.0373) -> (79.9688, 77.8902)
  line L562 (79.9688, 77.8902) -> (79.9017, 77.7503)
  line L563 (79.9017, 77.7503) -> (79.8214, 77.6185)
  line L564 (79.8214, 77.6185) -> (79.6261, 77.3817)
  line L565 (79.6261, 77.3817) -> (79.3894, 77.1863)
  line L566 (79.3894, 77.1863) -> (79.2574, 77.1061)
  line L567 (79.2574, 77.1061) -> (79.1176, 77.0387)
  line L568 (79.1176, 77.0387) -> (78.9705, 76.985)
  line L569 (78.9705, 76.985) -> (78.8172, 76.9455)
  line L570 (78.8172, 76.9455) -> (78.6583, 76.9212)
  line L571 (78.6583, 76.9212) -> (78.4947, 76.9131)
  line L572 (78.4947, 76.9131) -> (78.331, 76.9212)
  line L573 (78.331, 76.9212) -> (78.1722, 76.9455)
  line L574 (78.1722, 76.9455) -> (78.0189, 76.985)
  line L575 (78.0189, 76.985) -> (77.8718, 77.0387)
  line L576 (77.8718, 77.0387) -> (77.7319, 77.1061)
  line L577 (77.7319, 77.1061) -> (77.6, 77.1863)
  line L578 (77.6, 77.1863) -> (77.3633, 77.3817)
  line L579 (77.3633, 77.3817) -> (77.168, 77.6185)
  line L580 (77.168, 77.6185) -> (77.0877, 77.7503)
  line L581 (77.0877, 77.7503) -> (77.0205, 77.8902)
  line L582 (77.0205, 77.8902) -> (76.9668, 78.0373)
  line L583 (76.9668, 78.0373) -> (76.9272, 78.1906)
  line L584 (76.9272, 78.1906) -> (76.9031, 78.3494)
  line L585 (76.9031, 78.3494) -> (76.8948, 78.513)
  line L586 (-80.0974, 78.5005) -> (-80.0891, 78.6641)
  line L587 (-80.0891, 78.6641) -> (-80.0648, 78.8229)
  line L588 (-80.0648, 78.8229) -> (-80.0253, 78.9762)
  line L589 (-80.0253, 78.9762) -> (-79.9716, 79.1232)
  line L590 (-79.9716, 79.1232) -> (-79.9043, 79.263)
  line L591 (-79.9043, 79.263) -> (-79.824, 79.395)
  line L592 (-79.824, 79.395) -> (-79.6286, 79.6318)
  line L593 (-79.6286, 79.6318) -> (-79.3918, 79.8272)
  line L594 (-79.3918, 79.8272) -> (-79.26, 79.9073)
  line L595 (-79.26, 79.9073) -> (-79.1201, 79.9748)
  line L596 (-79.1201, 79.9748) -> (-78.973, 80.0285)
  line L597 (-78.973, 80.0285) -> (-78.8197, 80.068)
  line L598 (-78.8197, 80.068) -> (-78.6609, 80.0923)
  line L599 (-78.6609, 80.0923) -> (-78.4973, 80.1005)
  line L600 (-78.4973, 80.1005) -> (-78.3336, 80.0923)
  line L601 (-78.3336, 80.0923) -> (-78.1748, 80.068)
  line L602 (-78.1748, 80.068) -> (-78.0215, 80.0285)
  line L603 (-78.0215, 80.0285) -> (-77.8746, 79.9748)
  line L604 (-77.8746, 79.9748) -> (-77.7347, 79.9073)
  line L605 (-77.7347, 79.9073) -> (-77.6028, 79.8272)
  line L606 (-77.6028, 79.8272) -> (-77.3659, 79.6318)
  line L607 (-77.3659, 79.6318) -> (-77.1706, 79.395)
  line L608 (-77.1706, 79.395) -> (-77.0905, 79.263)
  line L609 (-77.0905, 79.263) -> (-77.0231, 79.1232)
  line L610 (-77.0231, 79.1232) -> (-76.9692, 78.9762)
  line L611 (-76.9692, 78.9762) -> (-76.9298, 78.8229)
  line L612 (-76.9298, 78.8229) -> (-76.9056, 78.6641)
  line L613 (-76.9056, 78.6641) -> (-76.8974, 78.5005)
  line L614 (-76.8974, 78.5005) -> (-76.9056, 78.3368)
  line L615 (-76.9056, 78.3368) -> (-76.9298, 78.178)
  line L616 (-76.9298, 78.178) -> (-76.9692, 78.0247)
  line L617 (-76.9692, 78.0247) -> (-77.0231, 77.8776)
  line L618 (-77.0231, 77.8776) -> (-77.0905, 77.7377)
  line L619 (-77.0905, 77.7377) -> (-77.1706, 77.6059)
  line L620 (-77.1706, 77.6059) -> (-77.3659, 77.3691)
  line L621 (-77.3659, 77.3691) -> (-77.6028, 77.1738)
  line L622 (-77.6028, 77.1738) -> (-77.7347, 77.0935)
  line L623 (-77.7347, 77.0935) -> (-77.8746, 77.0261)
  line L624 (-77.8746, 77.0261) -> (-78.0215, 76.9724)
  line L625 (-78.0215, 76.9724) -> (-78.1748, 76.9329)
  line L626 (-78.1748, 76.9329) -> (-78.3336, 76.9087)
  line L627 (-78.3336, 76.9087) -> (-78.4973, 76.9004)
  line L628 (-78.4973, 76.9004) -> (-78.6609, 76.9087)
  line L629 (-78.6609, 76.9087) -> (-78.8197, 76.9329)
  line L630 (-78.8197, 76.9329) -> (-78.973, 76.9724)
  line L631 (-78.973, 76.9724) -> (-79.1201, 77.0261)
  line L632 (-79.1201, 77.0261) -> (-79.26, 77.0935)
  line L633 (-79.26, 77.0935) -> (-79.3918, 77.1738)
  line L634 (-79.3918, 77.1738) -> (-79.6286, 77.3691)
  line L635 (-79.6286, 77.3691) -> (-79.824, 77.6059)
  line L636 (-79.824, 77.6059) -> (-79.9043, 77.7377)
  line L637 (-79.9043, 77.7377) -> (-79.9716, 77.8776)
  line L638 (-79.9716, 77.8776) -> (-80.0253, 78.0247)
  line L639 (-80.0253, 78.0247) -> (-80.0648, 78.178)
  line L640 (-80.0648, 78.178) -> (-80.0891, 78.3368)
  line L641 (-80.0891, 78.3368) -> (-80.0974, 78.5005)
  line L642 (-80.0974, -78.5041) -> (-80.0891, -78.3404)
  line L643 (-80.0891, -78.3404) -> (-80.0648, -78.1816)
  line L644 (-80.0648, -78.1816) -> (-80.0253, -78.0283)
  line L645 (-80.0253, -78.0283) -> (-79.9716, -77.8812)
  line L646 (-79.9716, -77.8812) -> (-79.9043, -77.7413)
  line L647 (-79.9043, -77.7413) -> (-79.824, -77.6097)
  line L648 (-79.824, -77.6097) -> (-79.6286, -77.3727)
  line L649 (-79.6286, -77.3727) -> (-79.3918, -77.1774)
  line L650 (-79.3918, -77.1774) -> (-79.26, -77.0971)
  line L651 (-79.26, -77.0971) -> (-79.1201, -77.0299)
  line L652 (-79.1201, -77.0299) -> (-78.973, -76.9762)
  line L653 (-78.973, -76.9762) -> (-78.8197, -76.9366)
  line L654 (-78.8197, -76.9366) -> (-78.6609, -76.9124)
  line L655 (-78.6609, -76.9124) -> (-78.4973, -76.9042)
  line L656 (-78.4973, -76.9042) -> (-78.3336, -76.9124)
  line L657 (-78.3336, -76.9124) -> (-78.1748, -76.9366)
  line L658 (-78.1748, -76.9366) -> (-78.0215, -76.9762)
  line L659 (-78.0215, -76.9762) -> (-77.8746, -77.0299)
  line L660 (-77.8746, -77.0299) -> (-77.7347, -77.0971)
  line L661 (-77.7347, -77.0971) -> (-77.6028, -77.1774)
  line L662 (-77.6028, -77.1774) -> (-77.3659, -77.3727)
  line L663 (-77.3659, -77.3727) -> (-77.1706, -77.6097)
  line L664 (-77.1706, -77.6097) -> (-77.0905, -77.7413)
  line L665 (-77.0905, -77.7413) -> (-77.0231, -77.8812)
  line L666 (-77.0231, -77.8812) -> (-76.9692, -78.0283)
  line L667 (-76.9692, -78.0283) -> (-76.9298, -78.1816)
  line L668 (-76.9298, -78.1816) -> (-76.9056, -78.3404)
  line L669 (-76.9056, -78.3404) -> (-76.8974, -78.5041)
  line L670 (-76.8974, -78.5041) -> (-76.9056, -78.6677)
  line L671 (-76.9056, -78.6677) -> (-76.9298, -78.8265)
  line L672 (-76.9298, -78.8265) -> (-76.9692, -78.9798)
  line L673 (-76.9692, -78.9798) -> (-77.0231, -79.127)
  line L674 (-77.0231, -79.127) -> (-77.0905, -79.2668)
  line L675 (-77.0905, -79.2668) -> (-77.1706, -79.3988)
  line L676 (-77.1706, -79.3988) -> (-77.3659, -79.6354)
  line L677 (-77.3659, -79.6354) -> (-77.6028, -79.8308)
  line L678 (-77.6028, -79.8308) -> (-77.7347, -79.9111)
  line L679 (-77.7347, -79.9111) -> (-77.8746, -79.9786)
  line L680 (-77.8746, -79.9786) -> (-78.0215, -80.0323)
  line L681 (-78.0215, -80.0323) -> (-78.1748, -80.0716)
  line L682 (-78.1748, -80.0716) -> (-78.3336, -80.0957)
  line L683 (-78.3336, -80.0957) -> (-78.4973, -80.104)
  line L684 (-78.4973, -80.104) -> (-78.6609, -80.0957)
  line L685 (-78.6609, -80.0957) -> (-78.8197, -80.0716)
  line L686 (-78.8197, -80.0716) -> (-78.973, -80.0323)
  line L687 (-78.973, -80.0323) -> (-79.1201, -79.9786)
  line L688 (-79.1201, -79.9786) -> (-79.26, -79.9111)
  line L689 (-79.26, -79.9111) -> (-79.3918, -79.8308)
  line L690 (-79.3918, -79.8308) -> (-79.6286, -79.6354)
  line L691 (-79.6286, -79.6354) -> (-79.824, -79.3988)
  line L692 (-79.824, -79.3988) -> (-79.9043, -79.2668)
  line L693 (-79.9043, -79.2668) -> (-79.9716, -79.127)
  line L694 (-79.9716, -79.127) -> (-80.0253, -78.9798)
  line L695 (-80.0253, -78.9798) -> (-80.0648, -78.8265)
  line L696 (-80.0648, -78.8265) -> (-80.0891, -78.6677)
  line L697 (-80.0891, -78.6677) -> (-80.0974, -78.5041)
  line L698 (76.8948, -78.4917) -> (76.9031, -78.328)
  line L699 (76.9031, -78.328) -> (76.9272, -78.1692)
  line L700 (76.9272, -78.1692) -> (76.9668, -78.0159)
  line L701 (76.9668, -78.0159) -> (77.0205, -77.8688)
  line L702 (77.0205, -77.8688) -> (77.0877, -77.7289)
  line L703 (77.0877, -77.7289) -> (77.168, -77.597)
  line L704 (77.168, -77.597) -> (77.3633, -77.3603)
  line L705 (77.3633, -77.3603) -> (77.6, -77.165)
  line L706 (77.6, -77.165) -> (77.7319, -77.0847)
  line L707 (77.7319, -77.0847) -> (77.8718, -77.0172)
  line L708 (77.8718, -77.0172) -> (78.0189, -76.9634)
  line L709 (78.0189, -76.9634) -> (78.1722, -76.9242)
  line L710 (78.1722, -76.9242) -> (78.331, -76.8997)
  line L711 (78.331, -76.8997) -> (78.4947, -76.8914)
  line L712 (78.4947, -76.8914) -> (78.6583, -76.8997)
  line L713 (78.6583, -76.8997) -> (78.8172, -76.9242)
  line L714 (78.8172, -76.9242) -> (78.9705, -76.9634)
  line L715 (78.9705, -76.9634) -> (79.1176, -77.0172)
  line L716 (79.1176, -77.0172) -> (79.2574, -77.0847)
  line L717 (79.2574, -77.0847) -> (79.3894, -77.165)
  line L718 (79.3894, -77.165) -> (79.6261, -77.3603)
  line L719 (79.6261, -77.3603) -> (79.8214, -77.597)
  line L720 (79.8214, -77.597) -> (79.9017, -77.7289)
  line L721 (79.9017, -77.7289) -> (79.9688, -77.8688)
  line L722 (79.9688, -77.8688) -> (80.0226, -78.0159)
  line L723 (80.0226, -78.0159) -> (80.0622, -78.1692)
  line L724 (80.0622, -78.1692) -> (80.0863, -78.328)
  line L725 (80.0863, -78.328) -> (80.0946, -78.4917)
  line L726 (80.0946, -78.4917) -> (80.0863, -78.655)
  line L727 (80.0863, -78.655) -> (80.0622, -78.8141)
  line L728 (80.0622, -78.8141) -> (80.0226, -78.9674)
  line L729 (80.0226, -78.9674) -> (79.9688, -79.1142)
  line L730 (79.9688, -79.1142) -> (79.9017, -79.2541)
  line L731 (79.9017, -79.2541) -> (79.8214, -79.386)
  line L732 (79.8214, -79.386) -> (79.6261, -79.623)
  line L733 (79.6261, -79.623) -> (79.3894, -79.8184)
  line L734 (79.3894, -79.8184) -> (79.2574, -79.8983)
  line L735 (79.2574, -79.8983) -> (79.1176, -79.9658)
  line L736 (79.1176, -79.9658) -> (78.9705, -80.0196)
  line L737 (78.9705, -80.0196) -> (78.8172, -80.0592)
  line L738 (78.8172, -80.0592) -> (78.6583, -80.0833)
  line L739 (78.6583, -80.0833) -> (78.4947, -80.0916)
  line L740 (78.4947, -80.0916) -> (78.331, -80.0833)
  line L741 (78.331, -80.0833) -> (78.1722, -80.0592)
  line L742 (78.1722, -80.0592) -> (78.0189, -80.0196)
  line L743 (78.0189, -80.0196) -> (77.8718, -79.9658)
  line L744 (77.8718, -79.9658) -> (77.7319, -79.8983)
  line L745 (77.7319, -79.8983) -> (77.6, -79.8184)
  line L746 (77.6, -79.8184) -> (77.3633, -79.623)
  line L747 (77.3633, -79.623) -> (77.168, -79.386)
  line L748 (77.168, -79.386) -> (77.0877, -79.2541)
  line L749 (77.0877, -79.2541) -> (77.0205, -79.1142)
  line L750 (77.0205, -79.1142) -> (76.9668, -78.9674)
  line L751 (76.9668, -78.9674) -> (76.9272, -78.8141)
  line L752 (76.9272, -78.8141) -> (76.9031, -78.655)
  line L753 (76.9031, -78.655) -> (76.8948, -78.4917)
  line L754 (-13.0005, -0.0003) -> (-12.9878, 0.2553)
  line L755 (-12.9878, 0.2553) -> (-12.9499, 0.5035)
  line L756 (-12.9499, 0.5035) -> (-12.8882, 0.7431)
  line L757 (-12.8882, 0.7431) -> (-12.8041, 0.9727)
  line L758 (-12.8041, 0.9727) -> (-12.6989, 1.1913)
  line L759 (-12.6989, 1.1913) -> (-12.5737, 1.3973)
  line L760 (-12.5737, 1.3973) -> (-12.4296, 1.5899)
  line L761 (-12.4296, 1.5899) -> (-12.2684, 1.7673)
  line L762 (-12.2684, 1.7673) -> (-12.0908, 1.9287)
  line L763 (-12.0908, 1.9287) -> (-11.8984, 2.0726)
  line L764 (-11.8984, 2.0726) -> (-11.6922, 2.1978)
  line L765 (-11.6922, 2.1978) -> (-11.4736, 2.303)
  line L766 (-11.4736, 2.303) -> (-11.244, 2.3873)
  line L767 (-11.244, 2.3873) -> (-11.0044, 2.4488)
  line L768 (-11.0044, 2.4488) -> (-10.7562, 2.4867)
  line L769 (-10.7562, 2.4867) -> (-10.5006, 2.4996)
  line L770 (-10.5006, 2.4996) -> (-10.2449, 2.4867)
  line L771 (-10.2449, 2.4867) -> (-9.9967, 2.4488)
  line L772 (-9.9967, 2.4488) -> (-9.7571, 2.3873)
  line L773 (-9.7571, 2.3873) -> (-9.5275, 2.303)
  line L774 (-9.5275, 2.303) -> (-9.3089, 2.1978)
  line L775 (-9.3089, 2.1978) -> (-9.1027, 2.0726)
  line L776 (-9.1027, 2.0726) -> (-8.9103, 1.9287)
  line L777 (-8.9103, 1.9287) -> (-8.7327, 1.7673)
  line L778 (-8.7327, 1.7673) -> (-8.5715, 1.5899)
  line L779 (-8.5715, 1.5899) -> (-8.4275, 1.3973)
  line L780 (-8.4275, 1.3973) -> (-8.3022, 1.1913)
  line L781 (-8.3022, 1.1913) -> (-8.197, 0.9727)
  line L782 (-8.197, 0.9727) -> (-8.1129, 0.7431)
  line L783 (-8.1129, 0.7431) -> (-8.0513, 0.5035)
  line L784 (-8.0513, 0.5035) -> (-8.0136, 0.2553)
  line L785 (-8.0136, 0.2553) -> (-8.0006, -0.0003)
  line L786 (-8.0006, -0.0003) -> (-8.0136, -0.256)
  line L787 (-8.0136, -0.256) -> (-8.0513, -0.5044)
  line L788 (-8.0513, -0.5044) -> (-8.1129, -0.7438)
  line L789 (-8.1129, -0.7438) -> (-8.197, -0.9736)
  line L790 (-8.197, -0.9736) -> (-8.3022, -1.192)
  line L791 (-8.3022, -1.192) -> (-8.4275, -1.398)
  line L792 (-8.4275, -1.398) -> (-8.5715, -1.5906)
  line L793 (-8.5715, -1.5906) -> (-8.7327, -1.768)
  line L794 (-8.7327, -1.768) -> (-8.9103, -1.9296)
  line L795 (-8.9103, -1.9296) -> (-9.1027, -2.0736)
  line L796 (-9.1027, -2.0736) -> (-9.3089, -2.1987)
  line L797 (-9.3089, -2.1987) -> (-9.5275, -2.3041)
  line L798 (-9.5275, -2.3041) -> (-9.7571, -2.3881)
  line L799 (-9.7571, -2.3881) -> (-9.9967, -2.4495)
  line L800 (-9.9967, -2.4495) -> (-10.2449, -2.4874)
  line L801 (-10.2449, -2.4874) -> (-10.5006, -2.5005)
  line L802 (-10.5006, -2.5005) -> (-10.7562, -2.4874)
  line L803 (-10.7562, -2.4874) -> (-11.0044, -2.4495)
  line L804 (-11.0044, -2.4495) -> (-11.244, -2.3881)
  line L805 (-11.244, -2.3881) -> (-11.4736, -2.3041)
  line L806 (-11.4736, -2.3041) -> (-11.6922, -2.1987)
  line L807 (-11.6922, -2.1987) -> (-11.8984, -2.0736)
  line L808 (-11.8984, -2.0736) -> (-12.0908, -1.9296)
  line L809 (-12.0908, -1.9296) -> (-12.2684, -1.768)
  line L810 (-12.2684, -1.768) -> (-12.4296, -1.5906)
  line L811 (-12.4296, -1.5906) -> (-12.5737, -1.398)
  line L812 (-12.5737, -1.398) -> (-12.6989, -1.192)
  line L813 (-12.6989, -1.192) -> (-12.8041, -0.9736)
  line L814 (-12.8041, -0.9736) -> (-12.8882, -0.7438)
  line L815 (-12.8882, -0.7438) -> (-12.9499, -0.5044)
  line L816 (-12.9499, -0.5044) -> (-12.9878, -0.256)
  line L817 (-12.9878, -0.256) -> (-13.0005, -0.0003)
  line L818 (7.998, -0.0003) -> (8.0111, 0.2553)
  line L819 (8.0111, 0.2553) -> (8.049, 0.5035)
  line L820 (8.049, 0.5035) -> (8.1104, 0.7431)
  line L821 (8.1104, 0.7431) -> (8.1944, 0.9727)
  line L822 (8.1944, 0.9727) -> (8.2998, 1.1913)
  line L823 (8.2998, 1.1913) -> (8.4252, 1.3973)
  line L824 (8.4252, 1.3973) -> (8.5689, 1.5899)
  line L825 (8.5689, 1.5899) -> (8.7305, 1.7673)
  line L826 (8.7305, 1.7673) -> (8.9079, 1.9287)
  line L827 (8.9079, 1.9287) -> (9.1005, 2.0726)
  line L828 (9.1005, 2.0726) -> (9.3065, 2.1978)
  line L829 (9.3065, 2.1978) -> (9.5249, 2.303)
  line L830 (9.5249, 2.303) -> (9.7547, 2.3873)
  line L831 (9.7547, 2.3873) -> (9.9941, 2.4488)
  line L832 (9.9941, 2.4488) -> (10.2425, 2.4867)
  line L833 (10.2425, 2.4867) -> (10.4982, 2.4996)
  line L834 (10.4982, 2.4996) -> (10.7538, 2.4867)
  line L835 (10.7538, 2.4867) -> (11.0018, 2.4488)
  line L836 (11.0018, 2.4488) -> (11.2416, 2.3873)
  line L837 (11.2416, 2.3873) -> (11.4714, 2.303)
  line L838 (11.4714, 2.303) -> (11.6898, 2.1978)
  line L839 (11.6898, 2.1978) -> (11.8958, 2.0726)
  line L840 (11.8958, 2.0726) -> (12.0884, 1.9287)
  line L841 (12.0884, 1.9287) -> (12.2658, 1.7673)
  line L842 (12.2658, 1.7673) -> (12.4271, 1.5899)
  line L843 (12.4271, 1.5899) -> (12.5711, 1.3973)
  line L844 (12.5711, 1.3973) -> (12.6965, 1.1913)
  line L845 (12.6965, 1.1913) -> (12.8015, 0.9727)
  line L846 (12.8015, 0.9727) -> (12.8856, 0.7431)
  line L847 (12.8856, 0.7431) -> (12.9473, 0.5035)
  line L848 (12.9473, 0.5035) -> (12.9852, 0.2553)
  line L849 (12.9852, 0.2553) -> (12.9983, -0.0003)
  line L850 (12.9983, -0.0003) -> (12.9852, -0.256)
  line L851 (12.9852, -0.256) -> (12.9473, -0.5044)
  line L852 (12.9473, -0.5044) -> (12.8856, -0.7438)
  line L853 (12.8856, -0.7438) -> (12.8015, -0.9736)
  line L854 (12.8015, -0.9736) -> (12.6965, -1.192)
  line L855 (12.6965, -1.192) -> (12.5711, -1.398)
  line L856 (12.5711, -1.398) -> (12.4271, -1.5906)
  line L857 (12.4271, -1.5906) -> (12.2658, -1.768)
  line L858 (12.2658, -1.768) -> (12.0884, -1.9296)
  line L859 (12.0884, -1.9296) -> (11.8958, -2.0736)
  line L860 (11.8958, -2.0736) -> (11.6898, -2.1987)
  line L861 (11.6898, -2.1987) -> (11.4714, -2.3041)
  line L862 (11.4714, -2.3041) -> (11.2416, -2.3881)
  line L863 (11.2416, -2.3881) -> (11.0018, -2.4495)
  line L864 (11.0018, -2.4495) -> (10.7538, -2.4874)
  line L865 (10.7538, -2.4874) -> (10.4982, -2.5005)
  line L866 (10.4982, -2.5005) -> (10.2425, -2.4874)
  line L867 (10.2425, -2.4874) -> (9.9941, -2.4495)
  line L868 (9.9941, -2.4495) -> (9.7547, -2.3881)
  line L869 (9.7547, -2.3881) -> (9.5249, -2.3041)
  line L870 (9.5249, -2.3041) -> (9.3065, -2.1987)
  line L871 (9.3065, -2.1987) -> (9.1005, -2.0736)
  line L872 (9.1005, -2.0736) -> (8.9079, -1.9296)
  line L873 (8.9079, -1.9296) -> (8.7305, -1.768)
  line L874 (8.7305, -1.768) -> (8.5689, -1.5906)
  line L875 (8.5689, -1.5906) -> (8.4252, -1.398)
  line L876 (8.4252, -1.398) -> (8.2998, -1.192)
  line L877 (8.2998, -1.192) -> (8.1944, -0.9736)
  line L878 (8.1944, -0.9736) -> (8.1104, -0.7438)
  line L879 (8.1104, -0.7438) -> (8.049, -0.5044)
  line L880 (8.049, -0.5044) -> (8.0111, -0.256)
  line L881 (8.0111, -0.256) -> (7.998, -0.0003)
  spline S3 degree 3 poles (-91.3883, -87.842) (-91.974, -88.4277) (-91.974, -89.3775) (-91.3883, -89.9635) knots 0 0 0 0 1 1 1 1
  line L882 (-91.3883, -87.842) -> (-91.974, -88.4277) construction
  line L883 (-91.974, -88.4277) -> (-91.974, -89.3775) construction
  line L884 (-91.974, -89.3775) -> (-91.3883, -89.9635) construction
  line L885 (-91.3883, -89.9635) -> (-89.9741, -91.3777)
  spline S4 degree 3 poles (-89.9741, -91.3777) (-89.3883, -91.9634) (-88.4384, -91.9634) (-87.8528, -91.3777) knots 2 2 2 2 3 3 3 3